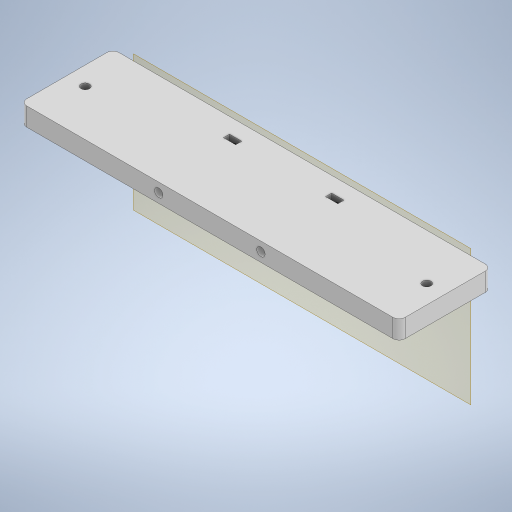
# Autodesk Inventor part: _battery_adt_2_
Saved by Autodesk Inventor 2024.3 (Build 283343000, 343)
## iProperties
Created: 2024-09-08
Part Number: _battery_adt_2_
Material: 일반
Document SubType Name: Modeling
Designer: gretc
Density: 1 g/cm^3
Appearance: 기본값
Author: gretc
Autodesk Inventor part; units mm, degrees
ref_plane "YZ Plane" through (0, 0, 0) normal (1, 0, 0) x (0, 1, 0)
ref_plane "XZ Plane" through (0, 0, 0) normal (0, 1, 0) x (-1, 0, 0)
ref_plane "XY Plane" through (0, 0, 0) normal (0, 0, 1) x (1, 0, 0)
ref_plane "작업 평면1" through (0, 0, 0) normal (0, 0, 1) x (1, 0, 0)
sketch "스케치1" plane through (0, 0, 0) normal (0, 0, 1) x (1, 0, 0)
  circle A0 centre (16.6, 17) radius 1.35 projected
  circle A1 centre (-16.6, 17) radius 1.35 projected
  line L0 (-49.8, -20) -> (49.8, -20) projected
  line L1 (49.8, -20) -> (49.8, 20) projected
  line L2 (49.8, 20) -> (-49.8, 20) projected
  line L3 (-49.8, 20) -> (-49.8, -20) projected
  circle A2 centre (40.6, -17) radius 1.35 projected
  circle A3 centre (30.7755, -17) radius 1.35 projected
  circle A4 centre (-40.6, -17) radius 1.35 projected
  circle A5 centre (-30.7755, -17) radius 1.35 projected
  line L4 (-49.8, 20) -> (-49.8, 14)
  line L5 (-49.8, 14) -> (49.8, 14)
  point P0 (0, 0)
  dimension "d0" = 6
  constraints: 4 end point, 2 point on line, 1 parallel
  measures "d0" distance of L2.end L4.end
extrude "돌출1" add sketch "스케치1" along normal blind 30 contours L3 L2 L1 L5
sketch "스케치2" plane through (-49.8, 20, 0) normal (0, 1, 0) x (1, 0, 0)
  line L0 (34.55, -30) -> (34.55, 0) projected
  line L1 (31.85, -30) -> (31.85, 0) projected
  line L2 (65.05, -30) -> (65.05, 0) projected
  line L3 (67.75, -30) -> (67.75, 0) projected
  line L4 (67.75, 0) -> (67.75, -6)
  line L5 (67.75, -6) -> (31.85, -6)
  line L6 (67.75, -6) -> (66.4, -6)
  line L7 (34.55, -6) -> (33.2, -6)
  line L8 (64.4, -5) -> (68.4, -5)
  line L9 (68.4, -5) -> (68.4, -7)
  line L10 (68.4, -7) -> (64.4, -7)
  line L11 (64.4, -7) -> (64.4, -5)
  line L12 (64.4, -5) -> (68.4, -7) construction
  line L13 (68.4, -5) -> (64.4, -7) construction
  line L14 (31.2, -5) -> (35.2, -5)
  line L15 (35.2, -5) -> (35.2, -7)
  line L16 (35.2, -7) -> (31.2, -7)
  line L17 (31.2, -7) -> (31.2, -5)
  line L18 (31.2, -5) -> (35.2, -7) construction
  line L19 (35.2, -5) -> (31.2, -7) construction
  point P0 (49.8, 0)
  point P1 (65.05, -6)
  dimension "d3" = 6
  dimension "d4" = 1.35
  dimension "d5" = 1.35
  dimension "d6" = 4
  dimension "d7" = 2
  dimension "d8" = 4
  dimension "d9" = 2
  constraints: 32 end point, 8 point on line, 4 midpoint, 4 parallel, 3 perpendicular, 2 coincident, 1 horizontal
  measures "d3" distance of L3.end L4.end
  measures "d4" distance of L6.start L6.end
  measures "d5" distance of L7.start L7.end
  measures "d6" distance of L8.start L8.end
  measures "d7" distance of L8.end L9.end
  measures "d8" distance of L14.start L14.end
  measures "d9" distance of L14.end L15.end
extrude "돌출2" cut sketch "스케치2" against normal up to surface (6 mm away)
sketch "스케치3" plane through (-49.8, 14, 0) normal (-1, 0, 0) x (0, 0, 1)
  line L0 (0, 6) -> (0, 0) projected
  line L1 (0, 0) -> (30, 0) projected
  line L2 (30, 6) -> (30, 0) projected
  line L3 (0, 6) -> (30, 6) projected
  point P0 (0, -14)
extrude "돌출3" add sketch "스케치3" along normal blind 11.7
sketch "스케치4" plane through (49.8, 14, 0) normal (1, 0, 0) x (0, 0, -1)
  line L0 (0, 0) -> (0, 6) projected
  line L1 (0, 6) -> (-30, 6) projected
  line L2 (-30, 0) -> (-30, 6) projected
  line L3 (0, 0) -> (-30, 0) projected
  point P0 (0, -14)
extrude "돌출4" add sketch "스케치4" along normal blind 11.7
sketch "스케치5" plane through (-61.5, 20, 30) normal (0, 1, 0) x (1, 0, 0)
  line L0 (42.9, 25) -> (46.9, 25) projected
  line L1 (46.9, 25) -> (46.9, 23) projected
  line L2 (46.9, 23) -> (42.9, 23) projected
  line L3 (42.9, 23) -> (42.9, 25) projected
  line L4 (80.1, 25) -> (80.1, 23) projected
  line L5 (80.1, 23) -> (76.1, 23) projected
  line L6 (76.1, 23) -> (76.1, 25) projected
  line L7 (76.1, 25) -> (80.1, 25) projected
  line L8 (0, 30) -> (123, 30) projected
  line L9 (0, 0) -> (0, 30) projected
  line L10 (0, 0) -> (123, 0) projected
  line L11 (123, 30) -> (123, 0) projected
  line L12 (0, 30) -> (3, 30)
  line L13 (3, 30) -> (3, 0)
  line L14 (123, 30) -> (120, 30)
  line L15 (120, 30) -> (120, 0)
  line L16 (0, 15) -> (123, 15)
  line L17 (3, 15) -> (3, 11)
  line L18 (3, 11) -> (123, 11)
  line L19 (3, 11) -> (3, 19)
  line L20 (3, 19) -> (9, 19)
  line L21 (9, 19) -> (9, 11)
  line L22 (9, 11) -> (3, 11)
  line L23 (120, 11) -> (120, 19)
  line L24 (120, 19) -> (114, 19)
  line L25 (114, 19) -> (114, 11)
  line L26 (114, 11) -> (120, 11)
  line L27 (3, 19) -> (9, 11)
  line L28 (3, 11) -> (9, 19)
  line L29 (114, 19) -> (120, 11)
  line L30 (114, 11) -> (120, 19)
  circle A0 centre (6, 15) radius 1.35
  circle A1 centre (117, 15) radius 1.35
  point P0 (61.5, 30)
  point P1 (120, 15)
  point P2 (9, 11)
  dimension "d16" = 3
  dimension "d17" = 3
  dimension "d18" = 4
  dimension "d19" = 8
  dimension "d20" = 6
  dimension "d21" = 6
  dimension "d24" = 2.7
  dimension "d25" = 2.7
  constraints: 38 end point, 13 point on line, 6 midpoint, 5 perpendicular, 4 parallel, 2 centre point
  measures "d16" distance of L8.start L12.end
  measures "d17" distance of L8.end L14.end
  measures "d18" distance of L17.start L17.end
  measures "d19" distance of L17.end L19.end
  measures "d20" distance of L19.end L20.end
  measures "d21" distance of L24.end L23.end
  measures "d24" diameter of A0
  measures "d25" diameter of A1
extrude "돌출6" cut sketch "스케치5" against normal up to surface (6 mm away) contours A0 L28 L27 | L27 L16 A0 | L16 L28 A0 | A1 L16 L30 | L30 L29 A1 | A0 L16 L28 | L16 A0 L27 | L27 A0 L28 | A1 L29 L16 | L29 L16 A1 | L30 A1 L16 | L29 A1 L30
fillet "모깎기1" radius 2 4 edges at (61.5, 17, 30) (61.5, 17, 0) (-61.5, 17, 0) (-61.5, 17, 30)
